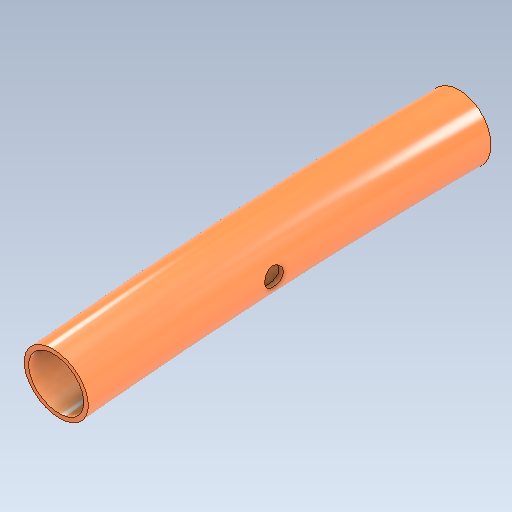
# Autodesk Inventor part: large_bearings
Saved by Autodesk Inventor 2021 (Build 250183000, 183)
## iProperties
Created: 2021-05-12
Part Number: large_bearings
Material: Polyurethane
Document SubType Name: Modeling
Density: 1.25 g/cm^3
Appearance: Generic
Autodesk Inventor part; units mm, degrees
ref_plane "YZ Plane" through (0, 0, 0) normal (1, 0, 0) x (0, 1, 0)
ref_plane "XZ Plane" through (0, 0, 0) normal (0, 1, 0) x (-1, 0, 0)
ref_plane "XY Plane" through (0, 0, 0) normal (0, 0, 1) x (1, 0, 0)
sketch "Sketch1" plane through (0, 0, 0) normal (1, 0, 0) x (0, 1, 0)
  circle A0 centre (0, 0) radius 1650
  dimension "d0" = 3300
  constraints: 1 centre point, 1 coincident
  measures "d0" diameter of A0
sketch "Sketch2" plane through (0, 0, 0) normal (0, 0, 1) x (1, 0, 0)
  circle A0 centre (0, 1650) radius 13.65
  circle A1 centre (0, 1650) radius 11.75
  line L0 (-19.11, 0) -> (19.11, 0) projected
  point P0 (0, 0)
  dimension "d1" = 1650
  dimension "d2" = 0
  dimension "d3" = 27.3
  dimension "d4" = 1.9
  constraints: 2 centre point, 1 coincident
  measures "d1" distance of point (0, 0) A0.centre
  measures "d2" horizontal distance of point (0, 0) A0.centre
  measures "d3" diameter of A0
  measures "d4" radial gap between concentric circles of A0 A1
revolve "Revolution1" add sketch "Sketch2" angle 6 about axis through (-10, 0, 0) along (1, 0, 0)
sketch "Sketch3" plane through (0, 0, 0) normal (1, 0, 0) x (0, 1, 0)
  line L0 (1637.311, 530.7226) -> (1398.8963, 530.7226)
  line L1 (1398.8963, 530.7226) -> (1398.8963, -338.3635)
  line L2 (1398.8963, -338.3635) -> (1637.311, -338.3635)
  line L3 (1637.311, -338.3635) -> (1637.311, 530.7226)
  point P0 (0, 0)
  constraints: 8 end point, 2 parallel, 1 horizontal, 1 perpendicular
extrude "Extrusion1" [suppressed]
sketch "Sketch4" plane through (0, 0, 0) normal (1, 0, 0) x (0, 1, 0)
  circle A0 centre (0, 0) radius 1650
  circle A1 centre (1647.385, 92.8591) radius 4
  dimension "d8" = 3300
  dimension "d9" = 8
  constraints: 1 centre point, 1 coincident, 3 other
  measures "d9" diameter of A1
extrude "Extrusion2" cut sketch "Sketch4" along normal mid plane 100 contours A1 A0 | A0 A1 picked at (1646.0721, 92.6243) picked at (1648.7179, 92.8591)
equation "\"d0\" = hoop_radius_large"
equation "\"d1\" = 0.5 * d0"
equation "\"d3\" = od"
equation "\"d4\" = t"
equation "\"d8\" = hoop_radius_large"
equation "\"hoop_radius_large\" = 3300"
equation "\"hoop_width_medium\" = 33.7"
equation "\"hoop_thickness_medium\" = 3.2"
equation "\"hoop_width_small\" = 25.4"
equation "\"hoop_bushing23_od\" = -2 * hoop_thickness_medium + hoop_width_medium + hoop_bushing23_radialInterference"
equation "\"hoop_bushing23_radialInterference\" = 0"
equation "\"hoop_bushing23_thickness\" = -hoop_width_small + hoop_bushing23_od - 2 * hoop_bushing23_radialInterference"
equation "\"od\" = hoop_bushing23_od"
equation "\"t\" = hoop_bushing23_thickness"
equation "\"hoop_angle_z\" = 45deg"
equation "\"hoop_bearing_length\" = 5deg"
equation "\"hoop_cable_diam\" = 5"
equation "\"hoop_cable_pulley_diam\" = 22"
equation "\"hoop_thickness_large\" = 4"
equation "\"hoop_thickness_small\" = 2"
equation "\"hoop_width_large\" = 51"
equation "\"hoop_bushing12_od\" = -2 * hoop_thickness_large + hoop_width_large + hoop_bushing12_radialInterference"
equation "\"hoop_bushing12_radialInterference\" = 0"
equation "\"hoop_bushing12_thickness\" = -hoop_width_medium + hoop_bushing12_od - 2 * hoop_bushing12_radialInterference"
equation "\"hoop_tabs_hole\" = 12"
equation "\"hoop_tabs_thickness\" = 6"
equation "\"rack_tooth_addendum\" = 5"
equation "\"rack_tooth_dedendum\" = 5"
equation "\"rack_tooth_thickness\" = 5"
equation "\"secure_arm_angle\" = 35deg"
equation "\"secure_arm_radii\" = 9"
equation "\"sm_varx_member_tolerance\" = 0"
equation "\"sm_varx_pinPlate_holeDiameter\" = 5"
equation "\"sm_varx_pinPlate_thickness\" = 5"
equation "\"sm_varx_squareBarThickness\" = 2.5"
equation "\"support_baseClamp_platformLengthBuffer\" = 35"
equation "\"support_baseClamp_platformThickness\" = 15"
equation "\"support_baseClamp_platformWidthBuffer\" = 0"
equation "\"support_baseClamp_sleeveHoleDiameter\" = 12"
equation "\"support_baseClamp_sleeveSweepTerminationAngle\" = 55deg"
equation "\"support_baseClamp_thickness\" = 8"
equation "\"support_frame_endHoleBuffer\" = 45"
equation "\"support_frame_squareBarFillet\" = 2"
equation "\"support_frame_squareBarThickness\" = 5"
equation "\"wheelchair_deployed_height\" = 914"
equation "\"wheelchair_deployed_length\" = 1067"
equation "\"wheelchair_deployed_width\" = 635"
equation "\"wheelchatir_pos_deploy_angle_0\" = 65deg"
equation "\"wheelchatir_pos_store_angle_0\" = 90deg"
equation "\"wheelchatir_pos_deploy_angle_1\" = 20deg"
equation "\"wheelchatir_pos_store_angle_1\" = 20deg"
body "Solid1"
